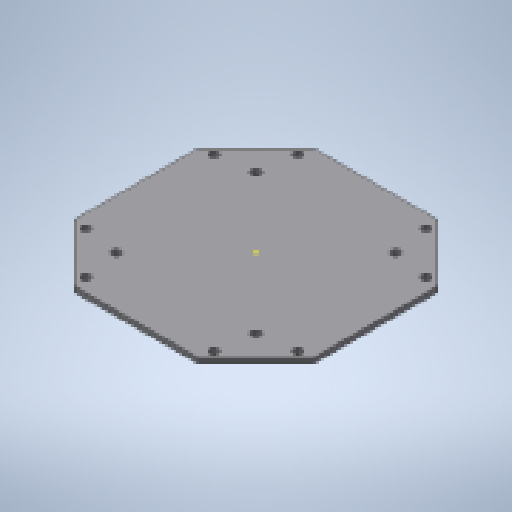
# Autodesk Inventor part: 上板
Saved by Autodesk Inventor 2025.2 (Build 292293000, 293)
## iProperties
Created: 2026-03-19
Part Number: 上板
Material: 常规
Document SubType Name: Modeling
Designer: BO‘S_SLAVE
Density: 1 g/cm^3
Appearance: 默认
Author: BO‘S_SLAVE
Autodesk Inventor part; units mm, degrees
ref_plane "YZ Plane" through (0, 0, 0) normal (1, 0, 0) x (0, 1, 0)
ref_plane "XZ Plane" through (0, 0, 0) normal (0, 1, 0) x (-1, 0, 0)
ref_plane "XY Plane" through (0, 0, 0) normal (0, 0, 1) x (1, 0, 0)
sketch "草图1" plane through (0, 0, 0) normal (0, 1, 0) x (-1, 0, 0)
  line L0 (35.3553, 35.3553) -> (-35.3553, 35.3553)
  line L1 (-35.3553, 35.3553) -> (-35.3553, -35.3553)
  line L2 (-35.3553, -35.3553) -> (35.3553, -35.3553)
  line L3 (35.3553, -35.3553) -> (35.3553, 35.3553)
  line L4 (35.3553, 35.3553) -> (-35.3553, -35.3553)
  line L5 (35.3553, -35.3553) -> (-35.3553, 35.3553)
  line L6 (-24.7487, 45.9619) -> (-45.9619, 24.7487)
  line L7 (-45.9619, -24.7487) -> (-24.7487, -45.9619)
  line L8 (24.7487, -45.9619) -> (45.9619, -24.7487)
  line L9 (45.9619, 24.7487) -> (24.7487, 45.9619)
  line L10 (24.7487, 45.9619) -> (-24.7487, 45.9619)
  line L11 (45.9619, 24.7487) -> (45.9619, -24.7487)
  line L12 (24.7487, -45.9619) -> (-24.7487, -45.9619)
  line L13 (-45.9619, -24.7487) -> (-45.9619, 24.7487)
  circle A0 centre (41.0122, 25.4558) radius 1.65
  circle A1 centre (27.5772, 27.5772) radius 1.65
  circle A2 centre (25.4558, 41.0122) radius 1.65
  circle A3 centre (-25.4558, 41.0122) radius 1.65
  circle A4 centre (-27.5772, 27.5772) radius 1.65
  circle A5 centre (-41.0122, 25.4558) radius 1.65
  circle A6 centre (-41.0122, -25.4558) radius 1.65
  circle A7 centre (-27.5772, -27.5772) radius 1.65
  circle A8 centre (-25.4558, -41.0122) radius 1.65
  circle A9 centre (25.4558, -41.0122) radius 1.65
  circle A10 centre (27.5772, -27.5772) radius 1.65
  circle A11 centre (41.0122, -25.4558) radius 1.65
  point P0 (0, 0)
  point P1 (0, 0)
  point P2 (-35.3553, -35.3553)
  point P3 (35.3553, -35.3553)
  dimension "d0" = 100
  dimension "d1" = 30
  dimension "d2" = 45
  dimension "d5" = 360
  dimension "d12" = 3.3
  dimension "d13" = 3
  dimension "d14" = 11
  dimension "d15" = 3.3
  dimension "d16" = 11
  dimension "d19" = 360
  constraints: 28 end point, 12 centre point, 6 perpendicular, 2 midpoint, 2 parallel, 1 coincident, 1 horizontal, 1 point on line, 1 symmetric about line, 43 other
  measures "d0" distance of L2.end L0.end
  measures "d1" distance of L6.start L6.end
  measures "d2" angle of L6 L1
  measures "d12" diameter of A0
  measures "d13" distance from line of L9 A0.centre
  measures "d14" distance from line of L4 A0.centre
  measures "d15" diameter of A1
  measures "d16" distance from line of L9 A1.centre
extrude "拉伸1" add sketch "草图1" along normal blind 3 contours L4 A1 L5 A4 L0 | L9 L11 L8 L3 | L3 L5 A10 L4 A1 | L0 L6 L10 L9 | L5 A4 L4 A7 L1 | L1 L7 L13 L6 | L8 L12 L7 L2 | L2 L4 A7 L5 A10
sketch "草图2" plane through (0, 3, 0) normal (0, 1, 0) x (1, 0, 0)
  line L0 (45.9619, -24.7487) -> (45.9619, 24.7487) projected
  line L1 (45.9619, 24.7487) -> (24.7487, 45.9619) projected
  line L2 (24.7487, 45.9619) -> (-24.7487, 45.9619) projected
  line L3 (-24.7487, 45.9619) -> (-45.9619, 24.7487) projected
  line L4 (-45.9619, 24.7487) -> (-45.9619, -24.7487) projected
  line L5 (-45.9619, -24.7487) -> (-24.7487, -45.9619) projected
  line L6 (-24.7487, -45.9619) -> (24.7487, -45.9619) projected
  line L7 (24.7487, -45.9619) -> (45.9619, -24.7487) projected
  circle A0 centre (27.5772, 27.5772) radius 1.65 projected
  circle A1 centre (-27.5772, 27.5772) radius 1.65 projected
  circle A2 centre (25.4558, -41.0122) radius 1.65 projected
  circle A3 centre (-25.4558, -41.0122) radius 1.65 projected
  circle A4 centre (-41.0122, 25.4558) radius 1.65 projected
  circle A5 centre (-41.0122, -25.4558) radius 1.65 projected
  circle A6 centre (25.4558, 41.0122) radius 1.65 projected
  circle A7 centre (-25.4558, 41.0122) radius 1.65 projected
  circle A8 centre (-27.5772, -27.5772) radius 1.65 projected
  circle A9 centre (41.0122, -25.4558) radius 1.65 projected
  circle A10 centre (41.0122, 25.4558) radius 1.65 projected
  circle A11 centre (27.5772, -27.5772) radius 1.65 projected
  line L8 (-45.9619, 0) -> (0, 0)
  line L9 (0, 0) -> (45.9619, 0)
  line L10 (0, 0) -> (0, 45.9619)
  line L11 (0, 0) -> (0, -45.9619)
  line L12 (-39.9619, -15) -> (-29.9619, -15)
  line L13 (-29.9619, -15) -> (-29.9619, 15)
  line L14 (-29.9619, 15) -> (-39.9619, 15)
  line L15 (-39.9619, 15) -> (-39.9619, -15)
  line L16 (-20, -16) -> (20, -16)
  line L17 (20, -16) -> (20, -8)
  line L18 (20, -8) -> (-20, -8)
  line L19 (-20, -8) -> (-20, -16)
  line L20 (39.9619, -15) -> (29.9619, -15)
  line L21 (29.9619, -15) -> (29.9619, 15)
  line L22 (29.9619, 15) -> (39.9619, 15)
  line L23 (39.9619, 15) -> (39.9619, -15)
  line L24 (-20, -35.9619) -> (20, -35.9619)
  line L25 (20, -35.9619) -> (20, -27.9619)
  line L26 (20, -27.9619) -> (-20, -27.9619)
  line L27 (-20, -27.9619) -> (-20, -35.9619)
  line L28 (-20, 16) -> (20, 16)
  line L29 (20, 16) -> (20, 8)
  line L30 (20, 8) -> (-20, 8)
  line L31 (-20, 8) -> (-20, 16)
  line L32 (-20, 35.9619) -> (20, 35.9619)
  line L33 (20, 35.9619) -> (20, 27.9619)
  line L34 (20, 27.9619) -> (-20, 27.9619)
  line L35 (-20, 27.9619) -> (-20, 35.9619)
  dimension "d21" = 30
  dimension "d22" = 10
  dimension "d23" = 6
  dimension "d24" = 15
  dimension "d25" = 8
  dimension "d27" = 8
  dimension "d29" = 40
  dimension "d30" = 20
  dimension "d31" = 8
  dimension "d32" = 40
  dimension "d33" = 20
  dimension "d34" = 10
  constraints: 56 end point, 12 symmetric about line, 6 parallel, 4 horizontal, 4 midpoint, 3 perpendicular
  measures "d21" distance between parallel lines of L14 L12
  measures "d22" distance between parallel lines of L13 L15
  measures "d23" distance between parallel lines of L4 L15
  measures "d24" distance between parallel lines of L8 L14
  measures "d25" distance between parallel lines of L16 L18
  measures "d27" distance between parallel lines of L8 L18
  measures "d29" distance between parallel lines of L17 L19
  measures "d30" distance between parallel lines of L11 L19
  measures "d31" distance between parallel lines of L24 L26
  measures "d32" distance between parallel lines of L25 L27
  measures "d33" distance between parallel lines of L11 L27
  measures "d34" distance between parallel lines of L6 L24
extrude "拉伸2" cut sketch "草图2" against normal through all contours L23 L20 L21 L9 | L9 L21 L22 L23 | L24 L27 L26 L11 | L11 L26 L25 L24 | L32 L33 L34 L10 | L10 L34 L35 L32 | L13 L12 L15 L8 | L8 L15 L14 L13 | L30 L31 L28 L10 | L10 L28 L29 L30 | L18 L17 L16 L11 | L11 L16 L19 L18
fillet "圆角1" radius 5 8 edges at (-39.9619, 1.5, 15) (-29.9619, 1.5, 15) (-39.9619, 1.5, -15) (-29.9619, 1.5, -15) (29.9619, 1.5, -15) (39.9619, 1.5, -15) (39.9619, 1.5, 15) (29.9619, 1.5, 15)
fillet "圆角2" radius 3 16 edges at (-20, 1.5, 35.9619) (-20, 1.5, 27.9619) (20, 1.5, 35.9619) (20, 1.5, 27.9619) (-20, 1.5, 16) (-20, 1.5, 8) (20, 1.5, 16) (20, 1.5, 8) (-20, 1.5, -8) (20, 1.5, -8) (-20, 1.5, -16) (20, 1.5, -16) (-20, 1.5, -27.9619) (-20, 1.5, -35.9619) (20, 1.5, -27.9619) (20, 1.5, -35.9619)
